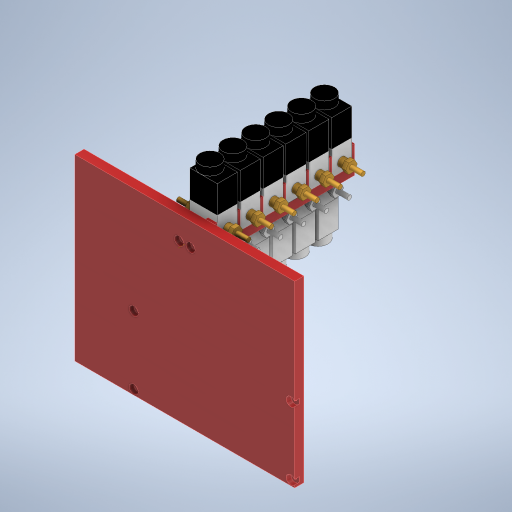
# Autodesk Inventor part: Montaje Valvulas
Saved by Autodesk Inventor 2024.2 (Build 282272000, 272)
## iProperties
Created: 2024-05-06
Part Number: Montaje Valvulas
Material: Generic
Document SubType Name: Modeling
Designer: jp.reyesf
Density: 1 g/cm^3
Appearance: Default
Author: jp.reyesf
Autodesk Inventor part; units mm, degrees
ref_plane "YZ Plane" through (0, 0, 0) normal (1, 0, 0) x (0, 1, 0)
ref_plane "XZ Plane" through (0, 0, 0) normal (0, 1, 0) x (-1, 0, 0)
ref_plane "XY Plane" through (0, 0, 0) normal (0, 0, 1) x (1, 0, 0)
sketch "Sketch1" plane through (0, 0, 0) normal (0, 1, 0) x (-1, 0, 0)
  line L0 (-15, 11) -> (15, 11)
  line L1 (15, 11) -> (15, -11)
  line L2 (15, -11) -> (-15, -11)
  line L3 (-15, -11) -> (-15, 11)
  line L4 (-15, 11) -> (15, -11) construction
  line L5 (15, 11) -> (-15, -11) construction
  line L6 (0, 0) -> (-10, 0)
  line L7 (-10, 7.5) -> (-10, -7.5) construction
  circle A0 centre (-10, 7.5) radius 2
  circle A1 centre (-10, -7.5) radius 2
  dimension "d0" = 22
  dimension "d1" = 30
  dimension "d2" = 15
  dimension "d3" = 5
  dimension "d4" = 4
  constraints: 16 end point, 3 midpoint, 2 centre point, 2 coincident, 2 horizontal, 2 parallel, 1 equal radius, 1 perpendicular, 1 vertical
  measures "d0" distance of L0.end L1.end
  measures "d1" distance of L1.end L2.end
  measures "d2" distance of L7.start L7.end
  measures "d3" distance between parallel lines of L7 L3
  measures "d4" diameter of A0
extrude "Extrusion1" add sketch "Sketch1" along normal blind 27
sketch "Sketch2" plane through (0, 27, 0) normal (0, 1, 0) x (1, 0, 0)
  line L0 (15, 11) -> (-15, 11) projected
  line L1 (-15, 11) -> (-15, -11) projected
  line L2 (-15, -11) -> (15, -11) projected
  line L3 (15, -11) -> (15, 11) projected
  circle A0 centre (10, 7.5) radius 2 projected
  circle A1 centre (10, -7.5) radius 2 projected
  point P0 (0, 0)
extrude "Extrusion2" add sketch "Sketch2" along normal blind 30 separate body contours L3 L2 L1 L0 | A0 | A1
sketch "Sketch3" plane through (0, 57, 0) normal (0, 1, 0) x (1, 0, 0)
  circle A0 centre (-4, 0) radius 11
  line L0 (15, 11) -> (-15, 11) projected
  line L1 (-15, 11) -> (-15, -11) projected
  line L2 (-15, -11) -> (15, -11) projected
  point P0 (0, 0)
  constraints: 3 tangent, 1 centre point
extrude "Extrusion3" add sketch "Sketch3" along normal blind 8.5 contours A0 bodies 2
sketch "Sketch4" plane through (15, 0, 11) normal (1, 0, 0) x (0, 0, -1)
  line L0 (11, 0) -> (11, 10) construction
  circle A0 centre (11, 10) radius 4.7
  dimension "d11" = 10
  dimension "d12" = 9.4
  constraints: 2 end point, 1 centre point, 1 coincident, 1 vertical
  measures "d11" distance of L0.start L0.end
  measures "d12" diameter of A0
extrude "Extrusion4" cut sketch "Sketch4" against normal blind 11.4 bodies 1
ref_plane "Work Plane1" through (0, 0, 11) normal (1, 0, 0) x (0, 0, -1)
mirror "Mirror1" about plane through (0, 0, 11) normal (1, 0, 0) of "Extrusion4" bodies 1
sketch "Sketch5" plane through (-15, 0, -11) normal (-1, 0, 0) x (0, 0, 1)
  circle A0 centre (11, 10) radius 4.7 projected
  point P0 (11, 0)
extrude "Extrusion5" add sketch "Sketch5" against normal up to surface (11.4 mm away) separate body
sketch "Sketch6" plane through (-15, 10, 0) normal (-1, 0, 0) x (0, 0, 1)
  circle A0 centre (0, 0) radius 4.7 projected
  point P0 (0, -10)
extrude "Extrusion6" add sketch "Sketch6" along normal blind 10.6 bodies 3
sketch "Sketch7" plane through (-25.6, 10, 0) normal (-1, 0, 0) x (0, 0, 1)
  circle A0 centre (0, 0) radius 4.7 projected
  line L0 (3.1754, 5.5) -> (6.3509, 0)
  line L1 (6.3509, 0) -> (3.1754, -5.5)
  line L2 (3.1754, -5.5) -> (-3.1754, -5.5)
  line L3 (-3.1754, -5.5) -> (-6.3509, 0)
  line L4 (-6.3509, 0) -> (-3.1754, 5.5)
  line L5 (-3.1754, 5.5) -> (3.1754, 5.5)
  circle A1 centre (0, 0) radius 2.4
  point P0 (0, -10)
  dimension "d19" = 11
  dimension "d22" = 4.8
  constraints: 12 end point, 2 coincident, 1 centre point, 1 horizontal, 13 other
  measures "d19" distance between parallel lines of L5 L2
  measures "d22" diameter of A1
extrude "Extrusion7" add sketch "Sketch7" against normal blind 4.6 contours A0 | L0 L1 L2 L3 L4 L5 | A1 bodies 3
extrude "Extrusion8" add sketch "Sketch7" along normal blind 12.7 contours A1 bodies 3
mirror "Mirror2" about plane through (0, 0, 11) normal (1, 0, 0) bodies 3
pattern_linear "Rectangular Pattern1" count 6 spacing 25 along (0, 0, -1) bodies 2 1 3
sketch "Sketch9" plane through (0, 0, 0) normal (0, -1, 0) x (1, 0, 0)
  line L0 (15, -11) -> (-15, -11) construction
  line L1 (15, 11) -> (15, -11) construction
  line L2 (-15, 11) -> (15, 11) construction
  line L3 (-15, -11) -> (-15, 11) construction
  circle A0 centre (10, -7.5) radius 2 construction
  circle A1 centre (10, 7.5) radius 2 construction
  line L4 (15, -36) -> (-15, -36) construction
  line L5 (15, -14) -> (15, -36) construction
  line L6 (-15, -14) -> (15, -14) construction
  line L7 (-15, -36) -> (-15, -14) construction
  circle A2 centre (10, -32.5) radius 2 construction
  circle A3 centre (10, -17.5) radius 2 construction
  line L8 (15, -61) -> (-15, -61) construction
  line L9 (15, -39) -> (15, -61) construction
  line L10 (-15, -39) -> (15, -39) construction
  line L11 (-15, -61) -> (-15, -39) construction
  circle A4 centre (10, -57.5) radius 2 construction
  circle A5 centre (10, -42.5) radius 2 construction
  line L12 (15, -86) -> (-15, -86) construction
  line L13 (15, -64) -> (15, -86) construction
  line L14 (-15, -64) -> (15, -64) construction
  line L15 (-15, -86) -> (-15, -64) construction
  circle A6 centre (10, -82.5) radius 2 construction
  circle A7 centre (10, -67.5) radius 2 construction
  line L16 (15, -111) -> (-15, -111) construction
  line L17 (15, -89) -> (15, -111) construction
  line L18 (-15, -89) -> (15, -89) construction
  line L19 (-15, -111) -> (-15, -89) construction
  circle A8 centre (10, -107.5) radius 2 construction
  circle A9 centre (10, -92.5) radius 2 construction
  line L20 (15, -136) -> (-15, -136) construction
  line L21 (15, -114) -> (15, -136) construction
  line L22 (-15, -114) -> (15, -114) construction
  line L23 (-15, -136) -> (-15, -114) construction
  circle A10 centre (10, -132.5) radius 2 construction
  circle A11 centre (10, -117.5) radius 2 construction
  circle A12 centre (10, 7.5) radius 2.1
  circle A13 centre (10, -7.5) radius 2.1
  circle A14 centre (10, -17.5) radius 2.1
  circle A15 centre (10, -32.5) radius 2.1
  circle A16 centre (10, -42.5) radius 2.1
  circle A17 centre (10, -57.5) radius 2.1
  circle A18 centre (10, -67.5) radius 2.1
  circle A19 centre (10, -82.5) radius 2.1
  circle A20 centre (10, -92.5) radius 2.1
  circle A21 centre (10, -107.5) radius 2.1
  circle A22 centre (10, -117.5) radius 2.1
  circle A23 centre (10, -132.5) radius 2.1
  line L24 (-30, 14) -> (15, 14)
  line L25 (15, 14) -> (15, -139)
  line L26 (15, -139) -> (-30, -139)
  line L27 (-30, -139) -> (-30, 14)
  line L28 (15, -11) -> (15, -10.3072) construction
  line L29 (15, 11) -> (15, -11) projected
  line L30 (-30, 14) -> (0, 14) construction
  line L31 (0, 14) -> (0, -8) construction
  line L32 (0, -8) -> (-30, -8) construction
  line L33 (-30, -8) -> (-30, 14) construction
  line L34 (-15, -11) -> (-15, 11) construction
  point P0 (0, -11)
  dimension "d35" = 0.1
  dimension "d36" = 3
  dimension "d83" = 3
  constraints: 18 end point, 12 centre point, 11 equal radius, 6 parallel, 2 horizontal, 2 perpendicular, 1 collinear, 1 midpoint, 1 point on line
  measures "d35" radial gap between concentric circles of A12 A1
  measures "d36" distance between parallel lines of L24 L2
  measures "d83" distance between parallel lines of L26 L20
extrude "Extrusion9" add sketch "Sketch9" along normal blind 10 separate body contours A12 | A13 | A14 | A15 | A16 | A17 | A18 | A19 | A20 | A21 | A22 | A23 | L24 L25 L26 L27
extrude "Extrusion12" cut sketch "Sketch9" along normal through all contours A12 | A13 | A14 | A15 | A16 | A17 | A18 | A19 | A20 | A21 | A22 | A23 bodies 1 4
sketch "Sketch10" plane through (0, -10, 0) normal (0, -1, 0) x (1, 0, 0)
  line L0 (-30, -139) -> (15, -139) projected
  line L1 (15, -139) -> (15, 14) projected
  line L2 (15, 14) -> (-30, 14) projected
  line L3 (-30, 14) -> (-30, -139) projected
  circle A0 centre (10, -132.5) radius 3.65
  circle A1 centre (10, -117.5) radius 3.65
  circle A2 centre (10, -107.5) radius 3.65
  circle A3 centre (10, -92.5) radius 3.65
  circle A4 centre (10, -82.5) radius 3.65
  circle A5 centre (10, -67.5) radius 3.65
  circle A6 centre (10, -57.5) radius 3.65
  circle A7 centre (10, -42.5) radius 3.65
  circle A8 centre (10, -32.5) radius 3.65
  circle A9 centre (10, -17.5) radius 3.65
  circle A10 centre (10, -7.5) radius 3.65
  circle A11 centre (10, 7.5) radius 3.65
  line L4 (-30, -139) -> (15, -139) projected
  circle A12 centre (10, 7.5) radius 2 projected
  circle A13 centre (10, -7.5) radius 2 projected
  circle A14 centre (10, -17.5) radius 2 projected
  circle A15 centre (10, -32.5) radius 2 projected
  circle A16 centre (10, -42.5) radius 2 projected
  circle A17 centre (10, -57.5) radius 2 projected
  circle A18 centre (10, -67.5) radius 2 projected
  circle A19 centre (10, -82.5) radius 2 projected
  circle A20 centre (10, -92.5) radius 2 projected
  circle A21 centre (10, -107.5) radius 2 projected
  circle A22 centre (10, -117.5) radius 2 projected
  circle A23 centre (10, -132.5) radius 2 projected
  point P0 (0, 0)
  dimension "d64" = 7.3
  constraints: 12 centre point, 12 concentric, 11 equal radius
  measures "d64" diameter of A0
extrude "Extrusion10" cut sketch "Sketch10" against normal blind 6 contours A0 | A1 | A2 | A3 | A4 | A5 | A6 | A7 | A8 | A9 | A10 | A11 | A12 | A13 | A14 | A15 | A16 | A17 | A18 | A19 | A20 | A21 | A22 | A23 bodies 4
sketch "Sketch12" plane through (-30, 0, 14) normal (0, 0, 1) x (1, 0, 0)
  line L0 (0, 0) -> (0, -10) projected
  line L1 (0, 0) -> (45, -10) construction
  circle A0 centre (16.25, -5) radius 2.5
  line L2 (16.25, -5) -> (28.75, -5) construction
  circle A1 centre (28.75, -5) radius 2.5
  point P0 (30, 0)
  point P1 (22.5, -5)
  dimension "d79" = 5
  dimension "d80" = 12.5
  constraints: 4 end point, 2 centre point, 2 coincident, 2 midpoint, 1 equal radius, 1 horizontal
  measures "d79" diameter of A0
  measures "d80" distance of L2.start L2.end
sketch "Sketch13" plane through (15, 0, 14) normal (1, 0, 0) x (0, 0, -1)
  line L0 (25.05, 20) -> (27.95, 20)
  line L1 (27.95, 20) -> (27.95, 0)
  line L2 (27.95, 0) -> (25.05, 0)
  line L3 (25.05, 0) -> (25.05, 20)
  line L4 (25, 0) -> (25, 27) projected
  line L5 (28, 0) -> (28, 27) projected
  point P0 (14, 0)
  dimension "d65" = 0.05
  dimension "d66" = 0.05
  dimension "d72" = 20
  constraints: 8 end point, 2 parallel, 1 horizontal, 1 perpendicular, 1 point on line
  measures "d65" distance between parallel lines of L4 L3
  measures "d66" distance between parallel lines of L5 L1
  measures "d72" distance between parallel lines of L0 L2
extrude "Extrusion13" add sketch "Sketch13" against normal up to surface (30 mm away) bodies 4
pattern_linear "Rectangular Pattern2" count 6 spacing 25 along (0, 0, -1) count 2 spacing 25 along (0, 0, 1) of "Extrusion13" bodies 4
chamfer "Chamfer2" distance 20 angle 45 7 edges at (-15, 20, -112.5) (-15, 20, -87.5) (-15, 20, -62.5) (-15, 20, -37.5) (-15, 20, -12.5) (-15, 20, 12.5) (-15, 20, -137.5)
pattern_circular "Circular Pattern2" count 2 over 360 about axis through (-7.5, -5, 14) along (0, 0, 1) of "Extrusion10", "Extrusion12", "Extrusion13", "Rectangular Pattern2", "Chamfer2" bodies 4
pattern_circular "Circular Pattern3" count 2 over 360 about axis through (-7.5, -5, 14) along (0, 0, 1) bodies 2 1 3 separate body
extrude "Extrusion14" cut sketch "Sketch12" against normal blind 10 bodies 4
sketch "Sketch14" plane through (-30, -10, 14) normal (0, 0, 1) x (1, 0, 0)
  line L0 (37, 75.5) -> (15, 75.5) projected
  line L1 (138.25, -160) -> (138.25, -86) construction
  line L2 (138.25, -86) -> (-33.25, -86) construction
  line L3 (-33.25, -86) -> (-33.25, -160) construction
  line L4 (-33.25, -160) -> (138.25, -160) construction
  circle A0 centre (138.25, -160) radius 1.65
  circle A1 centre (138.25, -86) radius 1.65
  circle A2 centre (-33.25, -160) radius 1.65
  circle A3 centre (-33.25, -86) radius 1.65
  line L5 (138.25, -160) -> (-33.25, -86) construction
  line L6 (142.5, -165.5) -> (142.5, -80.5) construction
  line L7 (142.5, -80.5) -> (-37.5, -80.5) construction
  line L8 (-37.5, -80.5) -> (-37.5, -165.5) construction
  line L9 (-37.5, -165.5) -> (142.5, -165.5) construction
  line L10 (142.5, -165.5) -> (-37.5, -80.5) construction
  line L11 (142.5, -80.5) -> (-37.5, -165.5) construction
  line L12 (-39.5, -165.5) -> (-39.5, -58.5) construction
  line L13 (-39.5, -58.5) -> (-97.5, -58.5) construction
  line L14 (-97.5, -58.5) -> (-97.5, -165.5) construction
  line L15 (-97.5, -165.5) -> (-39.5, -165.5) construction
  circle A4 centre (16.25, 5) radius 2.5 projected
  circle A5 centre (28.75, 5) radius 2.5 projected
  circle A6 centre (28.75, 5) radius 1.65
  circle A7 centre (16.25, 5) radius 1.65
  line L16 (68.3, 22.4) -> (68.3, 17.6) projected
  line L17 (0, 10) -> (0, 0) projected
  line L18 (168.3, 5) -> (28.75, 5) construction
  line L19 (-97.5, 30) -> (142.5, 30)
  line L20 (142.5, 30) -> (142.5, -165.5)
  line L21 (142.5, -165.5) -> (-97.5, -165.5)
  line L22 (-97.5, -165.5) -> (-97.5, 30)
  line L23 (45, 30) -> (35, 30) projected
  line L24 (8, -65.5) -> (30, -65.5) projected
  line L25 (28.75, 5) -> (16.25, 5)
  line L26 (45, 0) -> (0, 0) projected
  line L27 (16.25, 5) -> (22.5, 5)
  line L28 (22.5, 30) -> (22.5, 5) construction
  point P0 (30, 10)
  point P1 (52.5, -123)
  point P2 (142.5, -123)
  dimension "d88" = 74
  dimension "d89" = 171.5
  dimension "d90" = 3.3
  dimension "d91" = 180
  dimension "d92" = 85
  dimension "d93" = 107
  dimension "d95" = 3.3
  dimension "d96" = 3.3
  dimension "d105" = 2
  dimension "d106" = 195.5
  dimension "d107" = 15
  dimension "d108" = 240
  dimension "d111" = 58
  constraints: 46 end point, 9 parallel, 6 centre point, 6 coincident, 6 midpoint, 5 collinear, 5 perpendicular, 4 horizontal, 3 equal radius, 1 vertical
  measures "d88" distance of L3.end L2.end
  measures "d89" distance of L2.end L1.end
  measures "d90" diameter of A0
  measures "d91" distance from line of L8 point (142.5, -123)
  measures "d92" distance of L7.end L8.end
  measures "d93" distance between parallel lines of L15 L13
  measures "d95" diameter of A6
  measures "d96" diameter of A7
  measures "d105" distance between parallel lines of L12 L8
  measures "d106" distance of L21.end L19.start
  measures "d107" distance between parallel lines of L24 L7
  measures "d108" distance of L19.start L19.end
  measures "d111" distance between parallel lines of L12 L14
extrude "Extrusion17" add sketch "Sketch14" along normal blind 10 contours L19 L20 L21 L22 bodies 4
sketch "Sketch16" plane through (-30, -10, 24) normal (0, 0, 1) x (1, 0, 0)
  line L0 (-97.5, -165.5) -> (142.5, -165.5) projected
  line L1 (142.5, -165.5) -> (142.5, 30) projected
  line L2 (142.5, 30) -> (-97.5, 30) projected
  line L3 (-97.5, 30) -> (-97.5, -165.5) projected
  circle A0 centre (28.75, 5) radius 2.5 projected
  circle A1 centre (138.25, -160) radius 1.65 projected
  circle A2 centre (138.25, -86) radius 1.65 projected
  circle A3 centre (-33.25, -160) radius 1.65 projected
  circle A4 centre (-33.25, -86) radius 1.65 projected
  circle A5 centre (16.25, 5) radius 2.5 projected
  circle A6 centre (-33.25, -160) radius 5
  circle A7 centre (138.25, -160) radius 5
  circle A8 centre (138.25, -86) radius 5
  circle A9 centre (-33.25, -86) radius 5
  circle A10 centre (16.25, 5) radius 5
  circle A11 centre (28.75, 5) radius 5
  point P0 (30, 10)
  dimension "d112" = 10
  constraints: 6 centre point, 5 equal radius
  measures "d112" diameter of A6
extrude "Extrusion18" cut sketch "Sketch16" against normal blind 5 contours A7 L1 | L1 A7 | A8 L1 | L1 A8 | A0 | A1 | A2 | A3 | A4 | A5 | A6 | A9 | A10 | A11 bodies 4
body "Solid6"
body "Solid8"
body "Solid11"
body "Solid14"
body "Solid17"
body "Solid20"
body "Solid7"
body "Solid10"
body "Solid13"
body "Solid16"
body "Solid19"
body "Solid9"
body "Solid12"
body "Solid15"
body "Solid18"
body "Solid21"
body "Solid48"
body "Solid53"
body "Solid47"
body "Solid52"
body "Solid46"
body "Solid51"
body "Solid45"
body "Solid50"
body "Solid44"
body "Solid49"
body "Solid42"
body "Solid41"
body "Solid43"
body "Solid54"
body "Solid55"
body "Solid56"
body "Solid57"
body "Solid58"
